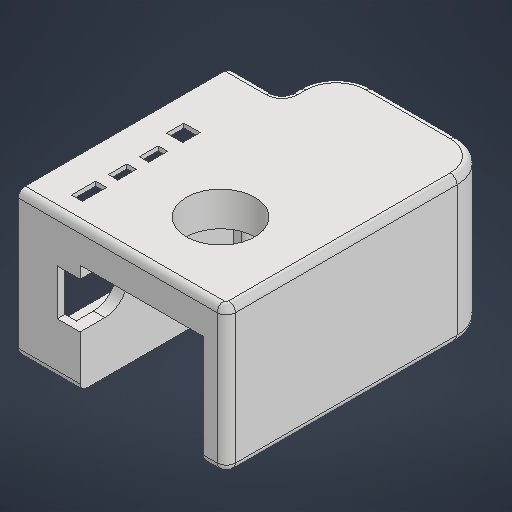
# Autodesk Inventor part: Part4
Saved by Autodesk Inventor 2025.3 (Build 293356030, 356C)
## iProperties
Created: 2025-09-19
Part Number: Part4
Material: Generic
Document SubType Name: Modeling
Designer: river
Density: 1 g/cm^3
Appearance: Default
Author: river
Autodesk Inventor part; units mm, degrees
ref_plane "YZ Plane" through (0, 0, 0) normal (1, 0, 0) x (0, 1, 0)
ref_plane "XZ Plane" through (0, 0, 0) normal (0, 1, 0) x (-1, 0, 0)
ref_plane "XY Plane" through (0, 0, 0) normal (0, 0, 1) x (1, 0, 0)
sketch "Sketch1" plane through (0, 0, 0) normal (0, 1, 0) x (-1, 0, 0)
  circle A0 centre (0, 0) radius 15
  line L0 (27.5, -33) -> (-26.5, -33)
  line L1 (-26.5, -33) -> (-26.5, 34)
  line L2 (-26.5, 34) -> (27.5, 34)
  line L3 (27.5, 34) -> (27.5, -33)
  line L4 (27.5, -15) -> (-26.5, -15) construction
  line L5 (15, -33) -> (15, 34) construction
  line L6 (0, 0) -> (0, -55.5) construction
  line L7 (15, -78) -> (-15, -78)
  line L8 (-15, -78) -> (-15, -33)
  line L9 (-15, -33) -> (15, -33)
  line L10 (15, -33) -> (15, -78)
  line L11 (15, -78) -> (-15, -33) construction
  line L12 (-15, -78) -> (15, -33) construction
  line L13 (0, -55.5) -> (0, -80.5) construction
  line L14 (11.5, -83) -> (-11.5, -83)
  line L15 (-11.5, -83) -> (-11.5, -78)
  line L16 (-11.5, -78) -> (11.5, -78)
  line L17 (11.5, -78) -> (11.5, -83)
  line L18 (11.5, -83) -> (-11.5, -78) construction
  line L19 (-11.5, -83) -> (11.5, -78) construction
  line L20 (-26.5, 34) -> (-36.5, 34)
  line L21 (-36.5, 34) -> (-36.5, -83)
  line L22 (-36.5, -83) -> (-11.5, -83)
  line L23 (27.5, 34) -> (32.5, 34)
  line L24 (32.5, 34) -> (32.5, -83)
  line L25 (32.5, -83) -> (11.5, -83)
  line L26 (21, -33) -> (21, -41)
  line L27 (21, -41) -> (15, -41)
  line L28 (-21, -33) -> (-21, -41)
  line L29 (-21, -41) -> (-15, -41)
  point P0 (15, -33)
  dimension "d0" = 30
  dimension "d1" = 54
  dimension "d2" = 67
  dimension "d3" = 18
  dimension "d4" = 12.5
  dimension "d6" = 45
  dimension "d7" = 5
  dimension "d8" = 23
  dimension "d9" = 10
  dimension "d10" = 5
  dimension "d20" = 8
  dimension "d21" = 6
  constraints: 60 end point, 9 perpendicular, 8 point on line, 6 horizontal, 6 parallel, 4 midpoint, 3 symmetric about line, 3 vertical, 2 tangent, 1 centre point, 1 coincident, 1 collinear
  measures "d0" diameter of A0
  measures "d1" distance of L0.start L0.end
  measures "d2" distance of L2.end L0.start
  measures "d3" distance between parallel lines of L0 L4
  measures "d4" distance between parallel lines of L5 L3
  measures "d6" distance of L7.end L8.end
  measures "d7" distance of L14.end L15.end
  measures "d8" distance of L14.start L14.end
  measures "d9" distance of L1.end L20.end
  measures "d10" distance of L2.end L23.end
  measures "d20" distance of L26.start L26.end
  measures "d21" distance between parallel lines of L10 L26
extrude "Extrusion1" add sketch "Sketch1" along normal blind 15
extrude "Extrusion2" add sketch "Sketch1" against normal blind 38 contours L3 L23 L24 L25 L17 L7 L10 L27 L26 L0 | L1 L0 L28 L29 L8 L7 L15 L22 L21 L20 | L14 L15 L7 L17
sketch "Sketch2" plane through (36.5, 15, -83) normal (0, 0, -1) x (-1, 0, 0)
  line L0 (51.5, -15) -> (21.5, -15) construction
  line L1 (51.5, -15) -> (51.5, -53) construction
  line L2 (21.5, -53) -> (51.5, -53) construction
  line L3 (21.5, -15) -> (21.5, -53) construction
  line L4 (21.5, -15) -> (51.5, -53) construction
  line L5 (21.5, -53) -> (51.5, -15) construction
  circle A0 centre (36.5, -34) radius 11.5
  point P0 (36.5, -15)
  dimension "d15" = 23
  constraints: 4 end point, 1 centre point, 1 midpoint
  measures "d15" diameter of A0
extrude "Extrusion3" cut sketch "Sketch2" against normal blind 38
extrude "Extrusion4" add sketch "Sketch1" against normal blind 10 from surface at -38 contours L3 L23 L24 L25 L17 L7 L10 L27 L26 L0 | L10 L7 L8 L0 | L1 L0 L28 L29 L8 L7 L15 L22 L21 L20 | L14 L15 L7 L17
sketch "Sketch3" plane through (-32.5, 15, -83) normal (-1, 0, 0) x (0, 0, 1)
  line L0 (117, -63) -> (117, 0) projected
  line L1 (0, 0) -> (117, 0) projected
  line L2 (0, -63) -> (0, 0) projected
  line L3 (0, -63) -> (117, -63) projected
  circle A0 centre (51.752, -54.7818) radius 1.35 projected
  circle A1 centre (109.752, -54.7818) radius 1.35 projected
  circle A2 centre (109.752, -5.7818) radius 1.35 projected
  circle A3 centre (51.752, -5.7818) radius 1.35 projected
  circle A4 centre (51.752, -5.7818) radius 3 projected
  circle A5 centre (109.752, -5.7818) radius 3 projected
  circle A6 centre (109.752, -54.7818) radius 3 projected
  circle A7 centre (51.752, -54.7818) radius 3 projected
  line L4 (31.252, -58.2818) -> (110.252, -58.2818) construction
  arc A8 (28.252, -55.2818) -> (31.252, -58.2818) centre (31.252, -55.2818) ccw construction
  line L5 (28.252, -5.2818) -> (28.252, -55.2818) construction
  arc A9 (31.252, -2.2818) -> (28.252, -5.2818) centre (31.252, -5.2818) ccw construction
  line L6 (110.252, -2.2818) -> (31.252, -2.2818) construction
  arc A10 (113.252, -5.2818) -> (110.252, -2.2818) centre (110.252, -5.2818) ccw construction
  line L7 (113.252, -55.2818) -> (113.252, -5.2818) construction
  arc A11 (110.252, -58.2818) -> (113.252, -55.2818) centre (110.252, -55.2818) ccw construction
  arc A12 (31.252, -1.8818) -> (27.852, -5.2818) centre (31.252, -5.2818) ccw
  line L8 (27.852, -5.2818) -> (27.852, -55.2818)
  arc A13 (27.852, -55.2818) -> (31.252, -58.6818) centre (31.252, -55.2818) ccw
  line L9 (31.252, -58.6818) -> (110.252, -58.6818)
  arc A14 (110.252, -58.6818) -> (113.652, -55.2818) centre (110.252, -55.2818) ccw
  line L10 (113.652, -55.2818) -> (113.652, -5.2818)
  arc A15 (113.652, -5.2818) -> (110.252, -1.8818) centre (110.252, -5.2818) ccw
  line L11 (110.252, -1.8818) -> (31.252, -1.8818)
  line L12 (53.7574, -1.8818) -> (53.7574, 0)
  line L13 (108.0983, -1.8818) -> (108.0983, 0)
  line L14 (117, 0) -> (0, 0) projected
  line L15 (23.6771, 0) -> (23.6771, -63)
  line L16 (23.6771, -3.7481) -> (28.2176, -3.7481)
  line L17 (23.6771, -56.367) -> (28.0299, -56.367)
  point P0 (31.1533, -58.8357)
  point P1 (110.1533, -58.8357)
  point P2 (110.1533, -8.8357)
  point P3 (31.1533, -8.8357)
  dimension "d23" = 0.4
  constraints: 18 end point, 10 point on circle, 8 point on line, 4 centre point, 4 perpendicular, 1 parallel, 7 other
  measures "d23" distance between parallel lines of L6 L11
extrude "Extrusion5" add sketch "Sketch3" along normal blind 22 contours L3 L15 L17 A13 L9 A14 L10 A15 L11 L13 L1 L0 | L12 L11 A12 L16 L15 L1
sketch "Sketch4" plane through (-32.5, -48, -83) normal (-1, 0, 0) x (0, 0, 1)
  circle A0 centre (51.752, 57.2182) radius 1.35 projected
  circle A1 centre (51.752, 57.2182) radius 3 projected
  circle A2 centre (109.752, 57.2182) radius 3 projected
  circle A3 centre (109.752, 57.2182) radius 1.35 projected
  circle A4 centre (51.752, 8.2182) radius 1.35 projected
  circle A5 centre (51.752, 8.2182) radius 3 projected
  circle A6 centre (109.752, 8.2182) radius 1.35 projected
  circle A7 centre (109.752, 8.2182) radius 3 projected
  point P0 (83, 48)
extrude "Extrusion6" add sketch "Sketch4" along normal blind 3
sketch "Sketch5" plane through (0, 15, 0) normal (0, 1, 0) x (1, 0, 0)
  line L0 (-32.5, 29.2426) -> (-54.5, 29.2426) projected
  line L1 (-32.5, 29.2426) -> (-32.5, -25.0983) projected
  line L2 (-32.5, -25.0983) -> (-54.5, -25.0983) projected
  line L3 (-54.5, 29.2426) -> (-54.5, -25.0983)
  line L4 (-40.6742, 5.1084) -> (-36.5345, 5.1084)
  line L5 (-36.5345, 5.1084) -> (-36.5345, 13.3208)
  line L6 (-36.5345, 13.3208) -> (-40.6742, 13.3208)
  line L7 (-40.6742, 13.3208) -> (-40.6742, 5.1084)
  line L8 (-40.6742, 5.1084) -> (-36.5345, 13.3208) construction
  line L9 (-36.5345, 5.1084) -> (-40.6742, 13.3208) construction
  line L10 (-40.6742, -8.4105) -> (-36.5345, -8.4105)
  line L11 (-36.5345, -8.4105) -> (-36.5345, -0.3447)
  line L12 (-36.5345, -0.3447) -> (-40.6742, -0.3447)
  line L13 (-40.6742, -0.3447) -> (-40.6742, -8.4105)
  line L14 (-40.6742, -8.4105) -> (-36.5345, -0.3447) construction
  line L15 (-36.5345, -8.4105) -> (-40.6742, -0.3447) construction
  line L16 (-40.9976, -24.2418) -> (-36.2112, -24.2418)
  line L17 (-36.2112, -24.2418) -> (-36.2112, -13.7372)
  line L18 (-36.2112, -13.7372) -> (-40.9976, -13.7372)
  line L19 (-40.9976, -13.7372) -> (-40.9976, -24.2418)
  line L20 (-40.9976, -24.2418) -> (-36.2112, -13.7372) construction
  line L21 (-36.2112, -24.2418) -> (-40.9976, -13.7372) construction
  line L22 (-43.6657, 19.9822) -> (-36.5345, 19.9822)
  line L23 (-36.5345, 19.9822) -> (-36.5345, 27.6033)
  line L24 (-36.5345, 27.6033) -> (-43.6657, 27.6033)
  line L25 (-43.6657, 27.6033) -> (-43.6657, 19.9822)
  line L26 (-43.6657, 19.9822) -> (-36.5345, 27.6033) construction
  line L27 (-36.5345, 19.9822) -> (-43.6657, 27.6033) construction
  point P0 (0, 0)
  point P1 (-38.6044, 9.2146)
  point P2 (-38.6044, -4.3776)
  point P3 (-38.6044, -18.9895)
  point P4 (-40.1001, 23.7927)
  constraints: 50 end point, 8 midpoint, 8 parallel, 5 perpendicular, 4 horizontal, 2 point on line
extrude "Extrusion7" add sketch "Sketch5" against normal up to surface (1.8818 mm away)
sketch "Sketch6" plane through (-32.5, 11.2519, -59.3229) normal (0, 0, -1) x (-1, 0, 0)
  line L0 (18.6624, -36.1361) -> (3.9019, -36.1361)
  line L1 (3.9019, -36.1361) -> (3.9019, -52.4625)
  line L2 (3.9019, -52.4625) -> (18.6624, -52.4625)
  line L3 (18.6624, -52.4625) -> (18.6624, -36.1361)
  line L4 (18.6624, -36.1361) -> (3.9019, -52.4625) construction
  line L5 (3.9019, -36.1361) -> (18.6624, -52.4625) construction
  line L6 (21.2933, -17.9508) -> (3.9019, -17.9508)
  line L7 (3.9019, -17.9508) -> (3.9019, -33.1185)
  line L8 (3.9019, -33.1185) -> (21.2933, -33.1185)
  line L9 (21.2933, -33.1185) -> (21.2933, -17.9508)
  line L10 (21.2933, -17.9508) -> (3.9019, -33.1185) construction
  line L11 (3.9019, -17.9508) -> (21.2933, -33.1185) construction
  line L12 (21.2994, -0.1915) -> (3.908, -0.1915)
  line L13 (3.908, -0.1915) -> (3.908, -15.0941)
  line L14 (3.908, -15.0941) -> (21.2994, -15.0941)
  line L15 (21.2994, -15.0941) -> (21.2994, -0.1915)
  line L16 (21.2994, -0.1915) -> (3.908, -15.0941) construction
  line L17 (3.908, -0.1915) -> (21.2994, -15.0941) construction
  line L18 (0, -59.2519) -> (0, 3.7481) projected
  line L19 (0, -52.6189) -> (22, -52.6189) projected
  line L20 (0, 0) -> (22, 0) projected
  line L21 (22, 0) -> (22, -52.6189)
  point P0 (-32.5, -11.2519)
  point P1 (11.2821, -44.2993)
  point P2 (12.5976, -25.5346)
  point P3 (12.6037, -7.6428)
  constraints: 38 end point, 6 midpoint, 6 parallel, 3 horizontal, 3 perpendicular, 1 vertical
extrude "Extrusion8" add sketch "Sketch6" against normal up to surface (4.5405 mm away)
fillet "Fillet1" radius 2 4 edges at (-32.5, 9.2182, 23.752) (-32.5, 9.2182, -34.248) (-32.5, -39.7818, 23.752) (-32.5, -39.7818, -34.248)
fillet "Fillet2" radius 4 1 edges at (-32.5, -16.5, -59.3229)
fillet "Fillet3" radius 16 2 edges at (36.5, -16.5, -83) (-32.5, -16.5, -83)
fillet "Fillet4" radius 4 1 edges at (36.5, -16.5, 34)
fillet "Fillet5" radius 3 11 edges at (-27.8137, 15, -78.3137) (-32.5, 15, -65.1614) (-33.6716, 15, -60.4944) (-45.5, 15, -59.3229) (31.8137, 15, -78.3137) (36.5, 15, -18.5) (35.3284, 15, 32.8284) (-11, 15, 34) (2, 15, -83) (-45.5, -48, -59.3229) (-41, -48, 34)
fillet "Fillet6" radius 3 10 edges at (-15, -19, -41) (-21, -24, -33) (15, -19, -41) (21, -24, -33) (-15, -43, -33) (15, -43, -33) (-15, -43, -41) (-21, -24, -41) (21, -24, -41) (15, -43, -41)
sketch "Sketch7" plane through (-32.5, -41.367, -54.7824) normal (-1, 0, 0) x (0, 0, 1)
  line L0 (85.4344, 51.0852) -> (85.4344, 1.0852) projected
  line L1 (77.9344, 16.0852) -> (92.9344, 16.0852)
  line L2 (92.9344, 16.0852) -> (92.9344, 36.0852)
  line L3 (92.9344, 36.0852) -> (77.9344, 36.0852)
  line L4 (77.9344, 36.0852) -> (77.9344, 16.0852)
  line L5 (77.9344, 16.0852) -> (92.9344, 36.0852) construction
  line L6 (92.9344, 16.0852) -> (77.9344, 36.0852) construction
  arc A0 (77.9344, 36.0852) -> (77.9344, 16.0852) centre (77.9344, 26.0852) ccw
  point P0 (54.7824, 41.367)
  point P1 (85.4344, 26.0852)
  dimension "d38" = 15
  dimension "d39" = 20
  constraints: 12 end point, 4 midpoint, 2 parallel, 2 point on circle, 1 centre point, 1 horizontal, 1 perpendicular
  measures "d38" distance of L3.end L2.end
  measures "d39" distance of L2.end L1.end
extrude "Extrusion9" cut sketch "Sketch7" along normal blind 5 and the other way blind 5
body "Solid1"
